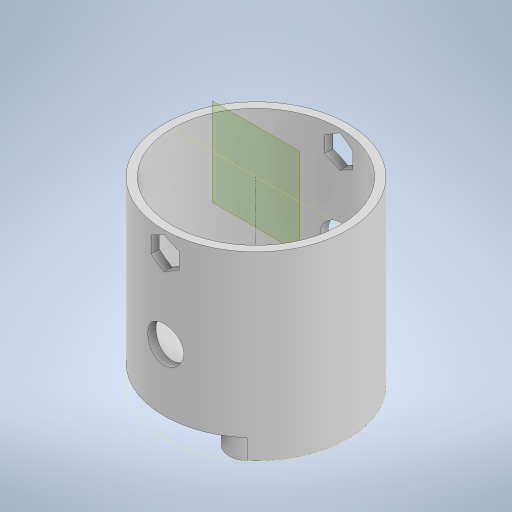
# Autodesk Inventor part: BasePotentiometer
Saved by Autodesk Inventor 2024 (Build 280153000, 153)
## iProperties
Created: 2023-10-09
Part Number: BasePotentiometer
Material: Generic
Document SubType Name: Modeling
Designer: Gibi500
Density: 1 g/cm^3
Appearance: Default
Author: Gibi500
## iProperties of the stored document BasePotentiometer_3DPrint.ipt
Created: 2023-10-09
Part Number: BasePotentiometer_3DPrint
Material: Generic
Document SubType Name: Modeling
Designer: Gibi500
Density: 1 g/cm^3
Appearance: Default
Author: Gibi500
Autodesk Inventor part; units mm, degrees
ref_plane "YZ Plane" through (0, 0, 0) normal (1, 0, 0) x (0, 1, 0)
ref_plane "XZ Plane" through (0, 0, 0) normal (0, 1, 0) x (-1, 0, 0)
ref_plane "XY Plane" through (0, 0, 0) normal (0, 0, 1) x (1, 0, 0)
sketch "Sketch1" plane through (0, 0, 0) normal (0, 1, 0) x (-1, 0, 0)
  circle A0 centre (0, 0) radius 23
  circle A1 centre (0, 0) radius 5.25
  dimension "d0" = 46
  dimension "d3" = 10.5
  constraints: 2 centre point, 2 coincident
  measures "d0" diameter of A0
  measures "d3" diameter of A1
extrude "Extrusion1" add sketch "Sketch1" along normal blind 2
sketch "Sketch2" plane through (0, 2, 0) normal (0, 1, 0) x (1, 0, 0)
  circle A0 centre (0, 0) radius 21
  circle A1 centre (0, 0) radius 23 projected
  line L0 (0, -23) -> (0, -21)
  line L1 (0, 21) -> (0, 23)
  dimension "d4" = 42
  constraints: 4 end point, 4 point on circle, 2 point on line, 1 centre point, 1 coincident, 1 vertical
  measures "d4" diameter of A0
extrude "Extrusion2" add sketch "Sketch2" along normal blind 38.3 contours A0 L1 A1 L0 | A0 L0 A1 L1
sketch "Sketch4" plane through (0, 0, 0) normal (0, -1, 0) x (1, 0, 0)
  circle A0 centre (0, 0) radius 5.25 projected
  arc A1 (6.9145, -15.5303) -> (7.1845, 15.4072) centre (0, 0) ccw construction
  arc A2 (9.3549, -21.0115) -> (9.7202, 20.8451) centre (0, 0) ccw
  arc A3 (4.4741, -10.049) -> (4.6488, 9.9694) centre (0, 0) ccw
  arc A4 (4.4741, -10.049) -> (9.3549, -21.0115) centre (6.9145, -15.5303) ccw
  arc A5 (9.7202, 20.8451) -> (4.6488, 9.9694) centre (7.1845, 15.4072) ccw
  line L0 (0, 0) -> (7.1845, 15.4072) construction
  line L1 (0, 0) -> (17, 0) construction
  line L2 (0, 0) -> (6.9145, -15.5303) construction
  line L3 (4.4741, -10.049) -> (9.3549, -21.0115)
  line L4 (4.6488, 9.9694) -> (9.7202, 20.8451)
  line L5 (6.9145, -15.5303) -> (10.1416, -13.6436) construction
  line L6 (0, 0) -> (3.2528, 0) construction
  line L7 (0, 0) -> (2, 0) construction
  dimension "d13" = 17
  dimension "d14" = 65
  dimension "d15" = 131
  dimension "d16" = 12
  constraints: 16 end point, 11 point on circle, 5 centre point, 4 tangent, 2 collinear, 2 point on line, 1 coincident, 1 equal length, 1 horizontal
  measures "d13" radius of A1
  measures "d14" angle of L1 L0
  measures "d15" angle of L2 L0
  measures "d16" diameter of A4
extrude "Extrusion4" add sketch "Sketch4" along normal blind 5 contours L3 A3 L4 A2
fillet "Fillet1" radius 5 4 edges at (4.4741, -2.5, -10.049) (9.3549, -2.5, -21.0115) (4.6488, -2.5, 9.9694) (9.7202, -2.5, 20.8451)
sketch "Sketch7" plane through (0, -5, 0) normal (0, -1, 0) x (1, 0, 0)
  arc A0 (14.8233, -17.586) -> (15.128, 17.3247) centre (0, 0) ccw projected
  line L0 (23, 0) -> (16, 0)
  circle A1 centre (16, 0) radius 3
  dimension "d35" = 7
  dimension "d36" = 6
  constraints: 2 end point, 1 centre point, 1 coincident, 1 horizontal, 1 point on circle
  measures "d35" distance of L0.start L0.end
  measures "d36" diameter of A1
extrude "Extrusion7" cut sketch "Sketch7" against normal blind 10
sketch "Sketch8" plane through (0, -5, 0) normal (0, -1, 0) x (1, 0, 0)
  circle A0 centre (0, 0) radius 23 construction
  line L0 (23, 0) -> (0, 0) construction
  line L1 (0, 0) -> (0, -23) construction
  constraints: 4 end point, 2 point on circle, 1 horizontal, 1 perpendicular
sketch "Sketch9" plane through (0, 0, 0) normal (0, 0, 1) x (1, 0, 0)
  line L0 (0, 0) -> (0, 40.3) construction
  line L1 (-21, 40.3) -> (21, 40.3) construction
  constraints: 2 end point, 1 midpoint
ref_plane "Work Plane2" through (0, 40.3, 0) normal (0, 0, -1) x (-1, 0, 0)
sketch "Sketch10" plane through (0, 40.3, 0) normal (0, 0, -1) x (-1, 0, 0)
  line L0 (-13.6647, -16.0448) -> (0, 0) construction
  line L1 (-21, 0) -> (21, 0) construction
  line L2 (0, 0) -> (0, -24.8) construction
  circle A0 centre (0, -24.8) radius 4.5
  point P0 (0, -40.3)
  dimension "d39" = 24.8
  dimension "d41" = 9
  constraints: 4 end point, 1 centre point, 1 coincident, 1 midpoint, 1 vertical
  measures "d39" distance of L0.end L2.end
  measures "d41" diameter of A0
extrude "Extrusion8" cut sketch "Sketch10" along normal mid plane 66.25
sketch "Sketch11" plane through (0, 40.3, 0) normal (0, 0, -1) x (-1, 0, 0)
  line L0 (0.1725, 0) -> (0.1725, -5.1914) construction
  line L1 (-3.5, -7.0207) -> (-3.5, -2.9793)
  line L2 (-3.5, -2.9793) -> (0, -0.9585)
  line L3 (0, -0.9585) -> (3.5, -2.9793)
  line L4 (3.5, -2.9793) -> (3.5, -7.0207)
  line L5 (3.5, -7.0207) -> (0, -9.0415)
  line L6 (0, -9.0415) -> (-3.5, -7.0207)
  point P0 (0, -40.3)
  point P1 (0, -5)
  constraints: 14 end point, 2 vertical, 13 other
extrude "Extrusion9" cut sketch "Sketch11" along normal mid plane 66.25
body "Solid1"
